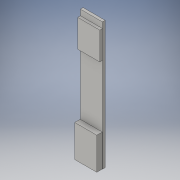
# Autodesk Inventor part: USW16T
Saved by Autodesk Inventor 2016 (Build 200138000, 138)
## iProperties
Created: 2015-12-06
Part Number: USW16T
Material: Generic
Document SubType Name: Modeling
Designer: Javier
Density: 1 g/cm^3
Appearance: Default
Author: Javier
Autodesk Inventor part; units mm, degrees
ref_plane "YZ Plane" through (0, 0, 0) normal (1, 0, 0) x (0, 1, 0)
ref_plane "XZ Plane" through (0, 0, 0) normal (0, 1, 0) x (-1, 0, 0)
sketch "Sketch1" plane through (0, 0, 0) normal (0, 0, 1) x (1, 0, 0)
  line L0 (-80, 463) -> (80, 463)
  line L1 (80, 463) -> (80, -463)
  line L2 (80, -463) -> (-80, -463)
  line L3 (-80, -463) -> (-80, 463)
  line L4 (0, 144.4625) -> (0, -193.675)
  line L5 (-174.625, 0) -> (185.7375, 0)
  point P0 (0, 0)
  dimension "d0" = 160
  dimension "d1" = 926
  constraints: 12 end point, 3 horizontal, 2 parallel, 2 vertical, 1 perpendicular, 2 other
  measures "d0" distance of L0.start L0.end
  measures "d1" distance of L0.end L1.end
extrude "Extrusion1" add sketch "Sketch1" along normal blind 20
ref_plane "Work Plane1" through (0, 0, 20) normal (0, 0, 1) x (1, 0, 0)
sketch "Sketch2" plane through (0, 0, 20) normal (0, 0, 1) x (1, 0, 0)
  line L0 (-78.9983, 421.7822) -> (81.0017, 421.7822)
  line L1 (81.0017, 421.7822) -> (81.0017, 221.7822)
  line L2 (81.0017, 221.7822) -> (-78.9983, 221.7822)
  line L3 (-78.9983, 221.7822) -> (-78.9983, 421.7822)
  point P0 (0, 0)
  dimension "d5" = 200
  dimension "d6" = 160
  constraints: 8 end point, 2 parallel, 1 horizontal, 1 perpendicular
  measures "d5" distance of L0.end L1.end
  measures "d6" distance of L0.start L0.end
extrude "Extrusion2" add sketch "Sketch2" along normal blind 20
sketch "Sketch3" plane through (0, 0, 20) normal (0, 0, 1) x (1, 0, 0)
  line L0 (-81.0461, -229.4574) -> (78.9539, -229.4574)
  line L1 (78.9539, -229.4574) -> (78.9539, -462.4574)
  line L2 (78.9539, -462.4574) -> (-81.0461, -462.4574)
  line L3 (-81.0461, -462.4574) -> (-81.0461, -229.4574)
  point P0 (0, 0)
  dimension "d9" = 233
  dimension "d10" = 160
  constraints: 8 end point, 2 parallel, 1 horizontal, 1 perpendicular
  measures "d9" distance of L0.end L1.end
  measures "d10" distance of L1.end L2.end
extrude "Extrusion3" add sketch "Sketch3" along normal blind 40
body "Solid1"
